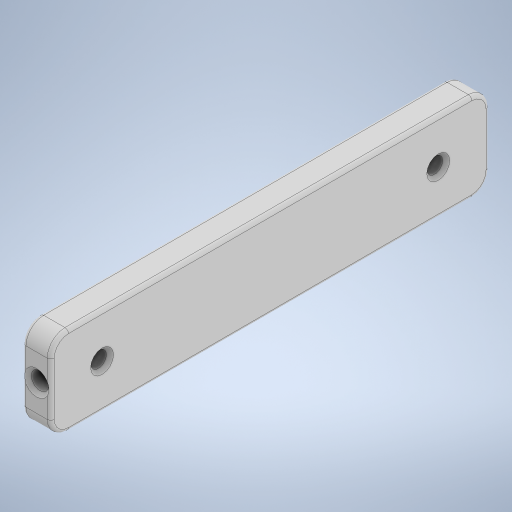
# Autodesk Inventor part: Camera_Adapter
Saved by Autodesk Inventor 2023 (Build 270158000, 158)
## iProperties
Created: 2023-05-30
Part Number: Camera_Adapter
Material: Generisch
Document SubType Name: Modeling
Designer: georg
Density: 1 g/cm^3
Appearance: Vorgabe
Author: georg
Autodesk Inventor part; units mm, degrees
ref_plane "YZ Plane" through (0, 0, 0) normal (1, 0, 0) x (0, 1, 0)
ref_plane "XZ Plane" through (0, 0, 0) normal (0, 1, 0) x (-1, 0, 0)
ref_plane "XY Plane" through (0, 0, 0) normal (0, 0, 1) x (1, 0, 0)
sketch "Skizze1" plane through (0, 0, 0) normal (1, 0, 0) x (0, 1, 0)
  line L0 (0, 0) -> (25, 0)
  line L1 (25, 0) -> (25, 124)
  line L2 (25, 124) -> (0, 124)
  line L3 (0, 124) -> (0, 0)
  dimension "d0" = 25
  dimension "d1" = 124
  constraints: 8 end point, 2 parallel, 1 horizontal, 1 perpendicular
  measures "d0" distance of L1.end L2.end
  measures "d1" distance of L0.end L1.end
extrude "Extrusion1" add sketch "Skizze1" along normal blind 8
fillet "Rundung1" radius 5 4 edges at (4, 25, 124) (4, 0, 124) (4, 25, 0) (4, 0, 0)
sketch "Skizze2" plane through (8, 0, 0) normal (1, 0, 0) x (0, 0, -1)
  circle A0 centre (-14.5, 12.5) radius 2.25
  circle A1 centre (-109.5, 12.5) radius 2.25
  line L0 (-124, 20) -> (-124, 5) projected
  line L1 (-5, 25) -> (-119, 25) projected
  point P0 (0, 0)
  dimension "d5" = 4.5
  dimension "d6" = 4.5
  dimension "d7" = 95
  dimension "d8" = 14.5
  dimension "d9" = 12.5
  dimension "d10" = 12.5
  constraints: 2 centre point
  measures "d5" diameter of A0
  measures "d6" diameter of A1
  measures "d7" distance of A0.centre A1.centre
  measures "d8" distance from line of L0 A1.centre
  measures "d9" distance from line of L1 A1.centre
  measures "d10" distance from line of L1 A0.centre
extrude "Extrusion2" cut sketch "Skizze2" against normal through all
sketch "Skizze3" plane through (0, 5, 0) normal (0, 0, -1) x (-1, 0, 0)
  circle A0 centre (-4, 7.5) radius 2.5
  line L0 (0, 20) -> (-8, 20) projected
  line L1 (-8, 0) -> (-8, 15) projected
  point P0 (0, -5)
  point P1 (-4, 20)
  dimension "d14" = 5
  dimension "d15" = 12.5
  dimension "d16" = 4
  constraints: 1 centre point, 1 midpoint
  measures "d14" diameter of A0
  measures "d15" distance of point (-4, 20) A0.centre
  measures "d16" distance from line of L1 A0.centre
extrude "Extrusion3" cut sketch "Skizze3" against normal blind 10
sketch "Skizze4" plane through (0, 5, 124) normal (0, 0, 1) x (1, 0, 0)
  circle A0 centre (4, 7.5) radius 2.5 projected
  point P0 (0, -5)
extrude "Extrusion4" cut sketch "Skizze4" against normal blind 10
chamfer "Fase1" distance 1 angle 45 2 edges at (1.5, 12.5, 124) (6.5, 12.5, 0)
fillet "Rundung3" radius 1 16 edges at (8, 23.5355, 1.4645) (8, 25, 62) (8, 23.5355, 122.5355) (8, 12.5, 124) (8, 1.4645, 122.5355) (8, 0, 62) (8, 1.4645, 1.4645) (8, 12.5, 0) (0, 23.5355, 1.4645) (0, 25, 62) (0, 23.5355, 122.5355) (0, 12.5, 124) (0, 1.4645, 122.5355) (0, 0, 62) (0, 1.4645, 1.4645) (0, 12.5, 0)
chamfer "Fase2" distance 1 angle 45 4 edges at (8, 12.5, 111.75) (8, 12.5, 16.75) (0, 12.5, 16.75) (0, 12.5, 111.75)
